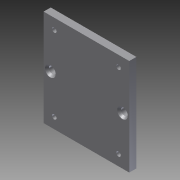
# Autodesk Inventor part: glass socket bottom
Saved by Autodesk Inventor 2011 (Build 150239000, 239)
## iProperties
Created: 2014-03-28
Part Number: glass socket bottom
Document SubType Name: Modeling
Designer: Devon
Density: 1 g/cm^3
Author: Devon
Autodesk Inventor part; units mm, degrees
ref_plane "YZ Plane" through (0, 0, 0) normal (1, 0, 0) x (0, 1, 0)
ref_plane "XZ Plane" through (0, 0, 0) normal (0, 1, 0) x (-1, 0, 0)
ref_plane "XY Plane" through (0, 0, 0) normal (0, 0, 1) x (1, 0, 0)
sketch "Sketch1" plane through (0, 0, 0) normal (0, 0, 1) x (1, 0, 0)
  line L0 (-57.7612, 63.8108) -> (18.4388, 63.8108)
  line L1 (18.4388, 63.8108) -> (18.4388, -22.1174)
  line L2 (18.4388, -22.1174) -> (-57.7612, -22.1174)
  line L3 (-57.7612, -22.1174) -> (-57.7612, 63.8108)
  line L4 (-57.7612, 63.8108) -> (-48.2362, 63.8108)
  line L5 (-48.2362, 63.8108) -> (-48.2362, 54.2858)
  line L6 (18.4388, 63.8108) -> (8.9138, 63.8108)
  line L7 (8.9138, 63.8108) -> (8.9138, 54.2858)
  line L8 (-57.7612, -22.1174) -> (-57.7612, -12.5924)
  line L9 (-57.7612, -12.5924) -> (-48.2362, -12.5924)
  circle A0 centre (-48.2362, 54.2858) radius 2.0193
  circle A1 centre (8.9138, 54.2858) radius 2.0193
  circle A2 centre (-48.2362, -12.5924) radius 2.0193
  circle A3 centre (8.9138, -12.5924) radius 2.0193
  circle A4 centre (-51.7612, 20.8467) radius 3.048
  circle A5 centre (12.4388, 20.8467) radius 3.048
  point P0 (0, 0)
  dimension "d0" = 76.2
  dimension "d1" = 85.9282
  dimension "d2" = 9.525
  dimension "d3" = 9.525
  dimension "d4" = 9.525
  dimension "d5" = 9.525
  dimension "d6" = 9.525
  dimension "d7" = 9.525
  dimension "d8" = 4.0386
  dimension "d9" = 4.0386
  dimension "d10" = 4.0386
  dimension "d11" = 4.0386
  dimension "d15" = 6.096
  dimension "d16" = 6.096
  constraints: 20 end point, 6 centre point, 4 perpendicular, 3 coincident, 3 point on line, 2 parallel, 1 horizontal
  measures "d0" distance of L1.end L2.end
  measures "d1" distance of L0.end L1.end
  measures "d2" distance of L0.start L4.end
  measures "d3" distance of L4.end L5.end
  measures "d4" distance of L0.end L6.end
  measures "d5" distance of L6.end L7.end
  measures "d6" distance of L2.end L8.end
  measures "d7" distance of L8.end L9.end
  measures "d8" diameter of A0
  measures "d9" diameter of A1
  measures "d10" diameter of A2
  measures "d11" diameter of A3
  measures "d15" diameter of A4
  measures "d16" diameter of A5
extrude "Extrusion1" add sketch "Sketch1" along normal blind 6.35
sketch "Sketch2" plane through (0, 0, 6.35) normal (0, 0, 1) x (1, 0, 0)
  circle A0 centre (12.4388, 20.8467) radius 3.048 projected
  circle A1 centre (-51.7612, 20.8467) radius 3.048 projected
  circle A2 centre (-51.7612, 20.8467) radius 3.048
  circle A3 centre (12.4388, 20.8467) radius 3.048
  point P0 (0, 0)
  constraints: 2 centre point, 2 coincident, 2 concentric
hole "Hole1" at (-51.7612, 20.8467, 6.35) at (12.4388, 20.8467, 6.35) direction (0, 0, -1) diameter 6.35 depth 25.4 tip angle 118 countersink diameter 9.525 countersink angle 82
body "Solid1"
